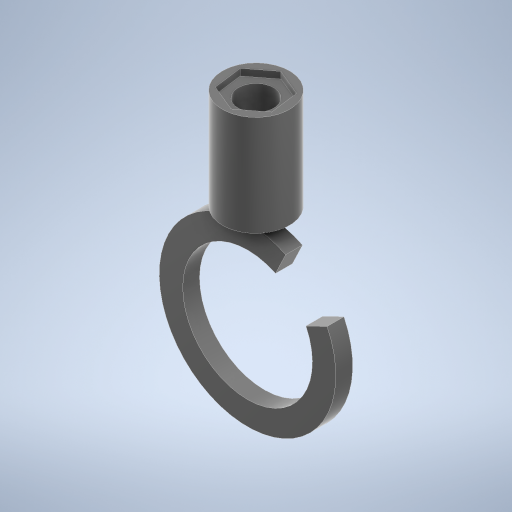
# Autodesk Inventor part: OriginNutipt
Saved by Autodesk Inventor 2023 (Build 270158000, 158)
## iProperties
Created: 2023-11-27
Part Number: OriginNutipt
Material: Thermoplastic Resin
Document SubType Name: Modeling
Designer: Mustapha
Density: 1.28 g/cm^3
Appearance: Smooth - Black
Mass: 1.92833 g
Surface Area: 14.994 cm^2
Volume: 1.50651 cm^3
Author: Mustapha
Autodesk Inventor part; units mm, degrees
ref_plane "YZ Plane" through (0, 0, 0) normal (1, 0, 0) x (0, 1, 0)
ref_plane "XZ Plane" through (0, 0, 0) normal (0, 1, 0) x (-1, 0, 0)
ref_plane "XY Plane" through (0, 0, 0) normal (0, 0, 1) x (1, 0, 0)
sketch "Sketch1" plane through (0, 0, 0) normal (0, 1, 0) x (-1, 0, 0)
  circle A0 centre (0, 0) radius 5
  dimension "d0" = 10
  constraints: 1 centre point, 1 coincident
  measures "d0" diameter of A0
extrude "Extrusion1" add sketch "Sketch1" along normal blind 15
sketch "Sketch2" plane through (0, 15, 0) normal (0, 1, 0) x (1, 0, 0)
  circle A0 centre (0, 0) radius 2.65
  dimension "d3" = 5.3
  constraints: 1 centre point, 1 coincident
  measures "d3" diameter of A0
extrude "Extrusion2" cut sketch "Sketch2" against normal blind 8
sketch "Sketch3" plane through (0, 0, 0) normal (0, -1, 0) x (1, 0, 0)
  line L0 (-1.6271, -1.2616) -> (1.6271, -1.2616)
  line L1 (1.6271, -1.2616) -> (1.6271, 1.2616)
  line L2 (1.6271, 1.2616) -> (-1.6271, 1.2616)
  line L3 (-1.6271, 1.2616) -> (-1.6271, -1.2616)
  circle A0 centre (0, 0) radius 5 projected
  line L4 (-1.6271, -1.2616) -> (1.6271, 1.2616) construction
  line L5 (1.6271, -1.2616) -> (-1.6271, 1.2616) construction
  constraints: 12 end point, 2 midpoint, 2 parallel, 1 horizontal, 1 perpendicular
extrude "Extrusion3" add sketch "Sketch3" along normal blind 5 contours L3 L2 L1 L0
sketch "Sketch4" plane through (-1.6271, 0, 1.2616) normal (0, 0, 1) x (1, 0, 0)
  circle A0 centre (1.6271, -14.7217) radius 13.1898
  arc A1 (5.8054, -5.9844) -> (10.354, -10.5216) centre (1.6271, -14.7217) ccw
  line L0 (1.6271, -14.7217) -> (13.5121, -9.0018)
  line L1 (1.6271, -14.7217) -> (7.5696, -2.2953)
  point P0 (1.6271, 0)
  point P1 (13.8416, -19.6992)
  point P2 (11.3121, -5.7679)
  point P3 (10.354, -10.5216)
  point P4 (7.3175, -2.8225)
  constraints: 5 point on circle, 4 end point, 2 centre point, 2 point on line, 1 coincident
extrude "Extrusion4" add sketch "Sketch4" against normal blind 2.512 contours A0 L1 A1 L0
sketch "Sketch5" plane through (0, 15, 0) normal (0, 1, 0) x (1, 0, 0)
  line L0 (-4, 1.6583) -> (-0.5639, 4.2933)
  line L1 (-0.5639, 4.2933) -> (3.4361, 2.6349)
  line L2 (3.4361, 2.6349) -> (4, -1.6583)
  line L3 (4, -1.6583) -> (0.5639, -4.2933)
  line L4 (0.5639, -4.2933) -> (-3.4361, -2.6349)
  line L5 (-3.4361, -2.6349) -> (-4, 1.6583)
  point P0 (0, 0)
  point P1 (0, 0)
  point P2 (-1.4361, -3.4641)
  dimension "d10" = 8
  dimension "d11" = 7.5
  constraints: 12 end point, 1 coincident, 1 midpoint, 13 other
  measures "d10" horizontal distance of L2.end L0.start
  measures "d11" distance from line of point (-1.436, -3.464) L1
extrude "Extrusion5" cut sketch "Sketch5" against normal blind 1
body "Solid1"
